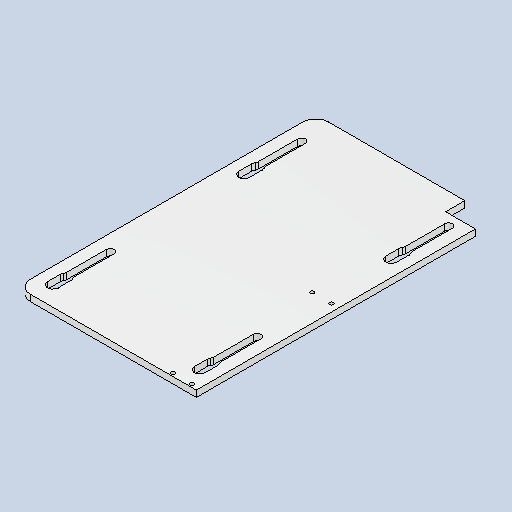
# Autodesk Inventor part: palp-desk
Saved by Autodesk Inventor 2026 (Build 300175050, 175E)
## iProperties
Created: 2025-12-08
Part Number: palp-desk
Material: Aluminum 6061
Document SubType Name: Modeling
Designer: kuzmin
Density: 2.7 g/cm^3
Appearance: Aluminum - Flat
Author: kuzmin
Autodesk Inventor part; units mm, degrees
ref_plane "YZ Plane" through (0, 0, 0) normal (1, 0, 0) x (0, 1, 0)
ref_plane "XZ Plane" through (0, 0, 0) normal (0, 1, 0) x (-1, 0, 0)
ref_plane "XY Plane" through (0, 0, 0) normal (0, 0, 1) x (1, 0, 0)
sketch "Sketch1" plane through (0, 0, 0) normal (0, 1, 0) x (-1, 0, 0)
  line L0 (210, 350) -> (-210, 350)
  line L1 (-210, 350) -> (-210, -350)
  line L2 (-210, -350) -> (210, -350)
  line L3 (210, -350) -> (210, 350)
  point P0 (0, 0)
  point P1 (210, 0)
  point P2 (0, -350)
  dimension "d0" = 420
  dimension "d1" = 700
  constraints: 8 end point, 2 midpoint, 2 parallel, 1 horizontal, 1 horizontal alignment, 1 perpendicular, 1 vertical alignment
  measures "d0" distance of L1.end L2.end
  measures "d1" distance of L2.end L0.start
extrude "Extrusion1" add sketch "Sketch1" along normal blind 15
sketch "Sketch2" plane through (0, 15, 0) normal (0, 1, 0) x (1, 0, 0)
  line L0 (-172.5, -279.5) -> (172.5, -279.5) construction
  line L1 (172.5, -279.5) -> (172.5, 169.5) construction
  line L2 (172.5, 169.5) -> (-172.5, 169.5) construction
  line L3 (-172.5, 169.5) -> (-172.5, -279.5) construction
  line L4 (-210, 350) -> (-210, -350) construction
  line L5 (210, 350) -> (-210, 350) construction
  line L6 (-210, -350) -> (210, -350) construction
  line L7 (-172.5, 144.5) -> (-172.5, 279.5) construction
  line L8 (-163.5, 144.5) -> (-163.5, 279.5)
  line L9 (-181.5, 279.5) -> (-181.5, 144.5)
  arc A0 (-181.5, 144.5) -> (-163.5, 144.5) centre (-172.5, 144.5) ccw
  arc A1 (-163.5, 279.5) -> (-181.5, 279.5) centre (-172.5, 279.5) ccw
  line L10 (-172.5, -169.5) -> (-172.5, -304.5) construction
  line L11 (-163.5, -169.5) -> (-163.5, -304.5)
  line L12 (-181.5, -304.5) -> (-181.5, -169.5)
  arc A2 (-163.5, -169.5) -> (-181.5, -169.5) centre (-172.5, -169.5) ccw
  arc A3 (-181.5, -304.5) -> (-163.5, -304.5) centre (-172.5, -304.5) ccw
  line L13 (172.5, -169.5) -> (172.5, -304.5) construction
  line L14 (181.5, -169.5) -> (181.5, -304.5)
  line L15 (163.5, -304.5) -> (163.5, -169.5)
  arc A4 (181.5, -169.5) -> (163.5, -169.5) centre (172.5, -169.5) ccw
  arc A5 (163.5, -304.5) -> (181.5, -304.5) centre (172.5, -304.5) ccw
  line L16 (172.5, 144.5) -> (172.5, 279.5) construction
  line L17 (181.5, 144.5) -> (181.5, 279.5)
  line L18 (163.5, 279.5) -> (163.5, 144.5)
  arc A6 (163.5, 144.5) -> (181.5, 144.5) centre (172.5, 144.5) ccw
  arc A7 (181.5, 279.5) -> (163.5, 279.5) centre (172.5, 279.5) ccw
  point P0 (0, 0)
  point P1 (0, 169.5)
  point P2 (-172.5, 212)
  point P3 (-172.5, -237)
  point P4 (172.5, -237)
  point P5 (172.5, 212)
  dimension "d5" = 180.5
  dimension "d7" = 18
  dimension "d9" = 25
  dimension "d10" = 110
  dimension "d11" = 110
  dimension "d12" = 25
  dimension "d46" = 345
  dimension "d47" = 449
  constraints: 40 end point, 16 point on circle, 16 tangent, 8 centre point, 8 point on line, 6 parallel, 5 midpoint, 4 horizontal alignment, 3 equal radius, 1 horizontal, 1 perpendicular, 1 vertical alignment
  measures "d5" distance between parallel lines of L5 L2
  measures "d7" distance between parallel lines of L8 L9
  measures "d9" distance of L2.end L7.start
  measures "d10" distance of L7.end L2.end
  measures "d11" distance of L10.start L0.start
  measures "d12" distance of L10.end L0.start
  measures "d46" distance of L1.end L2.end
  measures "d47" distance of L0.end L1.end
extrude "Extrusion2" cut sketch "Sketch2" against normal blind 15
fillet "Fillet1" radius 30 2 edges at (-210, 7.5, 350) (-210, 7.5, -350)
sketch "Sketch3" plane through (0, 15, 0) normal (0, 1, 0) x (1, 0, 0)
  line L0 (147.5, -342.5) -> (192.5, -342.5) construction
  line L1 (147.5, -15.5) -> (192.5, -15.5) construction
  line L2 (147.5, 342.5) -> (192.5, 342.5) construction
  line L3 (-180, -350) -> (210, -350) construction
  line L4 (210, -350) -> (210, 350) projected
  point P0 (0, 0)
  dimension "d17" = 45
  dimension "d18" = 327
  dimension "d19" = 358
  dimension "d48" = 147.5
  dimension "d49" = 15.5
  constraints: 6 coincident, 6 end point, 4 vertical alignment, 3 horizontal
  measures "d17" distance of L0.start L0.end
  measures "d18" distance between parallel lines of L0 L1
  measures "d19" distance from line of point (147.5, 342.5) L1
  measures "d48" horizontal distance of point (147.5, -15.5) point (0, 0)
  measures "d49" vertical distance of point (147.5, -15.5) point (0, 0)
hole "Hole1" at (147.5, 15, 342.5) at (192.5, 15, 342.5) at (147.5, 15, 15.5) at (192.5, 15, 15.5) at (147.5, 15, -342.5) at (192.5, 15, -342.5) direction (0, -1, 0) diameter 9 end through all
sketch "Sketch4" plane through (0, 15, 0) normal (0, 1, 0) x (1, 0, 0)
  line L0 (210, 305) -> (140, 305)
  line L1 (140, 305) -> (140, 350)
  line L2 (210, 350) -> (-180, 350) projected
  line L3 (210, -350) -> (210, 350) projected
  point P0 (0, 0)
  point P1 (210, 285)
  dimension "d29" = 45
  dimension "d50" = 140
  constraints: 4 end point, 3 point on line, 1 horizontal, 1 perpendicular
  measures "d29" distance between parallel lines of L2 L0
  measures "d50" distance from line of L1 point (0, 0)
extrude "Extrusion3" cut sketch "Sketch4" against normal through all
sketch "Sketch5" plane through (0, 15, 0) normal (0, 1, 0) x (1, 0, 0)
  arc A0 (-163.5, -169.5) -> (-181.5, -169.5) centre (-172.5, -169.5) ccw projected
  line L0 (-163.5, -169.5) -> (-163.5, -304.5) projected
  arc A1 (-181.5, -304.5) -> (-163.5, -304.5) centre (-172.5, -304.5) ccw projected
  line L1 (-181.5, -304.5) -> (-181.5, -169.5) projected
  arc A2 (181.5, -169.5) -> (163.5, -169.5) centre (172.5, -169.5) ccw projected
  line L2 (181.5, -169.5) -> (181.5, -304.5) projected
  arc A3 (163.5, -304.5) -> (181.5, -304.5) centre (172.5, -304.5) ccw projected
  line L3 (163.5, -304.5) -> (163.5, -169.5) projected
  line L4 (-181.5, 144.5) -> (-181.5, 279.5) projected
  arc A4 (-163.5, 279.5) -> (-181.5, 279.5) centre (-172.5, 279.5) ccw projected
  line L5 (-163.5, 279.5) -> (-163.5, 144.5) projected
  arc A5 (-181.5, 144.5) -> (-163.5, 144.5) centre (-172.5, 144.5) ccw projected
  line L6 (163.5, 144.5) -> (163.5, 279.5) projected
  arc A6 (181.5, 279.5) -> (163.5, 279.5) centre (172.5, 279.5) ccw projected
  line L7 (181.5, 279.5) -> (181.5, 144.5) projected
  arc A7 (163.5, 144.5) -> (181.5, 144.5) centre (172.5, 144.5) ccw projected
  circle A8 centre (147.5, -342.5) radius 4.5 projected
  circle A9 centre (192.5, -342.5) radius 4.5 projected
  circle A10 centre (147.5, -15.5) radius 4.5 projected
  circle A11 centre (192.5, -15.5) radius 4.5 projected
  line L8 (140, 350) -> (-180, 350) projected
  arc A12 (-180, 350) -> (-210, 320) centre (-180, 320) ccw projected
  line L9 (-210, 320) -> (-210, -320) projected
  arc A13 (-210, -320) -> (-180, -350) centre (-180, -320) ccw projected
  line L10 (-180, -350) -> (210, -350) projected
  line L11 (210, -350) -> (210, 305) projected
  line L12 (210, 305) -> (140, 305) projected
  line L13 (140, 305) -> (140, 350) projected
  line L14 (-172.5, -304.5) -> (-172.5, -274.5) construction
  line L15 (-160, -304.5) -> (-160, -274.5)
  line L16 (-185, -274.5) -> (-185, -304.5)
  arc A14 (-185, -304.5) -> (-160, -304.5) centre (-172.5, -304.5) ccw
  arc A15 (-160, -274.5) -> (-185, -274.5) centre (-172.5, -274.5) ccw
  line L17 (172.5, -304.5) -> (172.5, -274.5) construction
  line L18 (185, -304.5) -> (185, -274.5)
  line L19 (160, -274.5) -> (160, -304.5)
  arc A16 (160, -304.5) -> (185, -304.5) centre (172.5, -304.5) ccw
  arc A17 (185, -274.5) -> (160, -274.5) centre (172.5, -274.5) ccw
  line L20 (172.5, 144.5) -> (172.5, 174.5) construction
  line L21 (185, 144.5) -> (185, 174.5)
  line L22 (160, 174.5) -> (160, 144.5)
  arc A18 (160, 144.5) -> (185, 144.5) centre (172.5, 144.5) ccw
  arc A19 (185, 174.5) -> (160, 174.5) centre (172.5, 174.5) ccw
  line L23 (-172.5, 144.5) -> (-172.5, 174.5) construction
  line L24 (-160, 144.5) -> (-160, 174.5)
  line L25 (-185, 174.5) -> (-185, 144.5)
  arc A20 (-185, 144.5) -> (-160, 144.5) centre (-172.5, 144.5) ccw
  arc A21 (-160, 174.5) -> (-185, 174.5) centre (-172.5, 174.5) ccw
  point P0 (0, 0)
  point P1 (-172.5, -289.5)
  point P2 (172.5, -289.5)
  point P3 (172.5, 159.5)
  point P4 (-172.5, 159.5)
  point P5 (163.5, -265.8253)
  point P6 (181.5, -265.8253)
  point P7 (163.5, 183.1747)
  point P8 (181.5, 183.1747)
  point P9 (-181.5, 183.1747)
  point P10 (-163.5, 183.1747)
  point P11 (-181.5, -265.8253)
  point P12 (-163.5, -265.8253)
  dimension "d35" = 25
  dimension "d36" = 30
  dimension "d37" = 30
  dimension "d38" = 30
  dimension "d39" = 30
  dimension "d40" = 25
  dimension "d41" = 25
  dimension "d42" = 25
  constraints: 32 end point, 16 point on circle, 16 tangent, 8 centre point, 6 parallel, 4 midpoint, 1 point on line, 1 vertical
  measures "d35" distance between parallel lines of L15 L16
  measures "d36" distance of L14.start L14.end
  measures "d37" distance of L23.start L23.end
  measures "d38" distance of L20.start L20.end
  measures "d39" distance of L17.start L17.end
  measures "d40" distance between parallel lines of L18 L19
  measures "d41" distance between parallel lines of L24 L25
  measures "d42" distance between parallel lines of L21 L22
extrude "Extrusion4" cut sketch "Sketch5" against normal through all contours A15 L15 A14 L16 L1 A1 L0 | A17 L18 A16 L19 L3 A3 L2 | A5 L5 A21 L24 A20 L25 L4 | A7 L7 A19 L21 A18 L22 L6
fillet "Fillet3" radius 10 8 edges at (163.5, 7.5, 265.8253) (181.5, 7.5, 265.8253) (163.5, 7.5, -183.1747) (181.5, 7.5, -183.1747) (-181.5, 7.5, -183.1747) (-163.5, 7.5, -183.1747) (-181.5, 7.5, 265.8253) (-163.5, 7.5, 265.8253)
equation "\"d0\" = width"
equation "\"d1\" = length"
equation "\"d7\" = slotdi"
equation "\"d9\" = slotb"
equation "\"d10\" = slota"
equation "\"d11\" = slota"
equation "\"d12\" = slotb"
equation "\"d35\" = slotaldi"
equation "\"d36\" = slotalign"
equation "\"d37\" = slotalign"
equation "\"d38\" = slotalign"
equation "\"d39\" = slotalign"
equation "\"d40\" = slotaldi"
equation "\"d41\" = slotaldi"
equation "\"d42\" = slotaldi"
equation "\"slota\" = 110"
equation "\"slotb\" = 25"
equation "\"slotdi\" = 18"
equation "\"slotalign\" = 30"
equation "\"slotaldi\" = 25"
equation "\"width\" = 420"
equation "\"length\" = 700"
body "Solid1"
